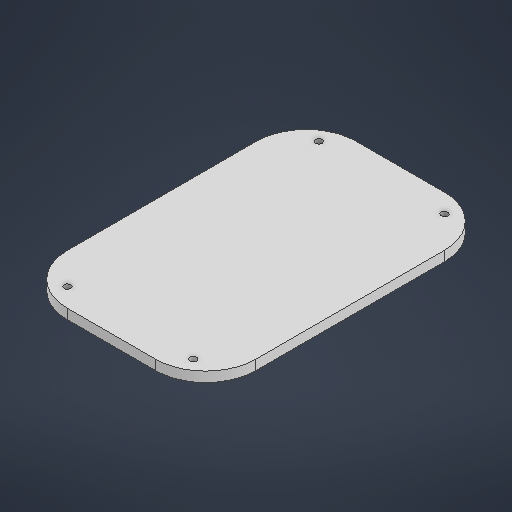
# Autodesk Inventor part: LiDAR_plate
Saved by Autodesk Inventor 2026 (Build 300175050, 175E)
## iProperties
Created: 2025-06-06
Part Number: LiDAR_plate
Material: Generic
Document SubType Name: Modeling
Designer: satom
Density: 1 g/cm^3
Appearance: Default
Author: satom
Autodesk Inventor part; units mm, degrees
ref_plane "YZ Plane" through (0, 0, 0) normal (1, 0, 0) x (0, 1, 0)
ref_plane "XZ Plane" through (0, 0, 0) normal (0, 1, 0) x (-1, 0, 0)
ref_plane "XY Plane" through (0, 0, 0) normal (0, 0, 1) x (1, 0, 0)
sketch "Sketch1" plane through (0, 0, 0) normal (0, 1, 0) x (-1, 0, 0)
  line L0 (-22.225, 73.025) -> (22.225, 73.025)
  line L1 (47.625, 47.625) -> (47.625, -47.625)
  line L2 (22.225, -73.025) -> (-22.225, -73.025)
  line L3 (-47.625, -47.625) -> (-47.625, 47.625)
  line L4 (-47.625, 73.025) -> (47.625, -73.025) construction
  line L5 (47.625, 73.025) -> (-47.625, -73.025) construction
  arc A0 (22.225, -73.025) -> (47.625, -47.625) centre (22.225, -47.625) ccw
  arc A1 (-47.625, -47.625) -> (-22.225, -73.025) centre (-22.225, -47.625) ccw
  arc A2 (-22.225, 73.025) -> (-47.625, 47.625) centre (-22.225, 47.625) ccw
  arc A3 (47.625, 47.625) -> (22.225, 73.025) centre (22.225, 47.625) ccw
  point P0 (0, 0)
  dimension "d11" = 95.25
  dimension "d12" = 146.05
  dimension "d13" = 25.4
  constraints: 12 end point, 8 point on circle, 8 point on line, 8 tangent, 4 centre point, 3 equal radius, 2 midpoint, 2 parallel, 1 horizontal, 1 perpendicular
  measures "d11" distance of L4.end L5.end
  measures "d12" distance of L5.start L4.end
  measures "d13" radius of A0
extrude "Extrusion1" add sketch "Sketch1" along normal blind 5
sketch "Sketch3" plane through (0, 5, 0) normal (0, 1, 0) x (1, 0, 0)
  circle A0 centre (-31.75, -63.5) radius 1.7
  line L0 (-47.625, 47.625) -> (-47.625, -47.625) construction
  line L1 (-47.625, 0) -> (47.625, 0) construction
  line L2 (47.625, -47.625) -> (47.625, 47.625) construction
  line L3 (0, -72.5867) -> (0, 73.025) construction
  line L4 (22.225, 73.025) -> (-22.225, 73.025) construction
  circle A1 centre (-31.75, 63.5) radius 1.7
  circle A2 centre (31.75, -63.5) radius 1.7
  circle A3 centre (31.75, 63.5) radius 1.7
  point P0 (0, 0)
  dimension "d14" = 3.4
  dimension "d15" = 63.5
  dimension "d16" = 31.75
  constraints: 4 centre point, 4 end point, 3 midpoint, 3 symmetric about line, 1 horizontal, 1 vertical, 3 other
  measures "d14" diameter of A0
  measures "d15" distance from line of L1 A0.centre
  measures "d16" distance from line of L3 A0.centre
extrude "Extrusion2" cut sketch "Sketch3" against normal through all
equation "\"d3\" = hardboard_thickness"
equation "\"d14\" = m3_clearance"
equation "\"m3_heat_set_insert\" = 4"
equation "\"m3_clearance\" = 3.4"
equation "\"m3_heat_set_depth\" = 7"
equation "\"robot_diameter\" = 354"
equation "\"hardboard_thickness\" = 5"
body "Solid1"
